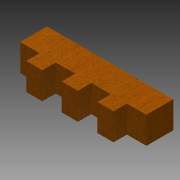
# Autodesk Inventor part: Separator
Saved by Autodesk Inventor 2014 SP1 (Build 180222100, 222)
## iProperties
Created: 2014-02-22
Part Number: Separator
Material: Wood
Document SubType Name: Modeling
Designer: tuleu
Density: 0.570257 g/cm^3
Appearance: Yellow Pine - Solid Natural Low Gloss
Author: tuleu
Autodesk Inventor part; units mm, degrees
ref_plane "YZ Plane" through (0, 0, 0) normal (1, 0, 0) x (0, 1, 0)
ref_plane "XZ Plane" through (0, 0, 0) normal (0, 1, 0) x (-1, 0, 0)
ref_plane "XY Plane" through (0, 0, 0) normal (0, 0, 1) x (1, 0, 0)
sketch "Sketch1" plane through (0, 0, 0) normal (0, 0, 1) x (1, 0, 0)
  line L0 (-45, 0) -> (-45, -40) construction
  line L1 (-68, -840) -> (-68, 0) construction
  line L2 (-98, 0) -> (-98, -840) construction
  line L3 (-121, -40) -> (-121, 0) construction
  line L4 (-151, 0) -> (-151, -40) construction
  line L5 (-174, -840) -> (-174, 0) construction
  line L6 (-15, -40) -> (-15, 0) construction
  line L7 (8, 0) -> (8, -840) construction
  line L8 (11, 2) -> (-18, 2)
  line L9 (-18, 2) -> (-18, -18)
  line L10 (-18, -18) -> (-42, -18)
  line L11 (-42, -18) -> (-42, 2)
  line L12 (-42, 2) -> (-71, 2)
  line L13 (-71, 2) -> (-71, -18)
  line L14 (-71, -18) -> (-95, -18)
  line L15 (-95, -18) -> (-95, 2)
  line L16 (-95, 2) -> (-124, 2)
  line L17 (-124, 2) -> (-124, -18)
  line L18 (-124, -18) -> (-148, -18)
  line L19 (-148, -18) -> (-148, 2)
  line L20 (-148, 2) -> (-177, 2)
  line L21 (-177, 2) -> (-177, 42)
  line L22 (-177, 42) -> (11, 42)
  line L23 (11, 42) -> (11, 2)
  point P0 (0, 0)
  dimension "d0" = 60
  dimension "d1" = 40
  dimension "d2" = 2
  dimension "d3" = 3
  dimension "d4" = 3
  dimension "d5" = 3
  dimension "d6" = 3
  dimension "d7" = 3
  dimension "d8" = 3
  dimension "d9" = 3
  dimension "d10" = 3
  constraints: 32 end point, 9 equal length, 5 collinear, 4 perpendicular, 2 vertical
  measures "d0" distance between parallel lines of L22 L10
  measures "d1" distance between parallel lines of L22 L8
  measures "d2" distance from line of point (0, 0) L8
  measures "d3" distance between parallel lines of L6 L9
  measures "d4" distance between parallel lines of L0 L11
  measures "d5" distance between parallel lines of L1 L13
  measures "d6" distance between parallel lines of L2 L15
  measures "d7" distance between parallel lines of L17 L3
  measures "d8" distance between parallel lines of L4 L19
  measures "d9" distance between parallel lines of L5 L21
  measures "d10" distance between parallel lines of L7 L23
extrude "Extrusion1" add sketch "Sketch1" against normal blind 40
body "Solid1"
